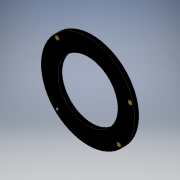
# Autodesk Inventor part: Neo_Cercle
Saved by Autodesk Inventor 2017 (Build 210142000, 142)
## iProperties
Created: 2018-11-03
Part Number: Neo_Cercle
Material: Generic
Document SubType Name: Modeling
Designer: ludov
Density: 1 g/cm^3
Appearance: Default
Author: ludov
Autodesk Inventor part; units mm, degrees
ref_plane "YZ Plane" through (0, 0, 0) normal (1, 0, 0) x (0, 1, 0)
ref_plane "XZ Plane" through (0, 0, 0) normal (0, 1, 0) x (-1, 0, 0)
ref_plane "XY Plane" through (0, 0, 0) normal (0, 0, 1) x (1, 0, 0)
sketch "Esquisse1" plane through (0, 0, 0) normal (0, 1, 0) x (-1, 0, 0)
  circle A0 centre (0, 0) radius 18.325
  dimension "d0" = 36.65
  constraints: 1 centre point, 1 coincident
  measures "d0" diameter of A0
extrude "Extrusion1" add sketch "Esquisse1" along normal blind 1.6
sketch "Esquisse2" plane through (0, 1.6, 0) normal (0, 1, 0) x (1, 0, 0)
  circle A0 centre (0, 0) radius 11.7
  dimension "d3" = 23.4
  constraints: 1 centre point, 1 coincident
  measures "d3" diameter of A0
hole "Perçage1" at (0, 1.6, 0) direction (0, -1, 0) diameter 23.4 end through all
sketch "Esquisse18" plane through (0, 1.6, 0) normal (0, 1, 0) x (1, 0, 0)
  line L0 (0, 0) -> (12.0738, 12.0738)
  line L1 (0, 0) -> (17.075, 0) construction
  circle A0 centre (12.0738, 12.0738) radius 0.8
  dimension "d116" = 17.075
  dimension "d117" = 45
  dimension "d118" = 1.6
  constraints: 4 end point, 1 centre point, 1 coincident, 1 equal length, 1 horizontal
  measures "d116" distance of L0.start L0.end
  measures "d117" angle of L1 L0
  measures "d118" diameter of A0
extrude "Extrusion14" add sketch "Esquisse18" along normal blind 0.05
sketch "Esquisse19" plane through (12.0738, 1.65, -12.0738) normal (0, 1, 0) x (1, 0, 0)
  circle A0 centre (0, 0) radius 0.45
  point P0 (-12.0738, -12.0738)
  dimension "d121" = 0.9
  constraints: 1 centre point
  measures "d121" diameter of A0
hole "Perçage2" at (12.0738, 1.65, -12.0738) direction (0, -1, 0) diameter 0.9 end through all
sketch "Esquisse20" plane through (0, 1.6, 0) normal (0, 1, 0) x (1, 0, 0)
  line L0 (0, 0) -> (16.4932, -4.4193)
  line L1 (0, 0) -> (17.075, 0) construction
  circle A0 centre (16.4932, -4.4193) radius 0.8
  dimension "d129" = 17.075
  dimension "d130" = 345
  dimension "d131" = 1.6
  constraints: 4 end point, 2 coincident, 1 centre point, 1 equal length, 1 horizontal
  measures "d129" distance of L0.start L0.end
  measures "d131" diameter of A0
extrude "Extrusion15" add sketch "Esquisse20" along normal blind 0.05
sketch "Esquisse21" plane through (16.4932, 1.65, 4.4193) normal (0, 1, 0) x (1, 0, 0)
  circle A0 centre (0, 0) radius 0.45
  point P0 (-16.4932, 4.4193)
  dimension "d134" = 0.9
  constraints: 1 centre point
  measures "d134" diameter of A0
hole "Perçage3" at (16.4932, 1.65, 4.4193) direction (0, -1, 0) diameter 0.9 end through all
sketch "Esquisse22" plane through (0, 1.6, 0) normal (0, 1, 0) x (1, 0, 0)
  line L0 (0, 0) -> (-12.0738, 12.0738)
  line L1 (0, 0) -> (17.075, 0) construction
  circle A0 centre (-12.0738, 12.0738) radius 0.8
  dimension "d142" = 17.075
  dimension "d143" = 135
  dimension "d144" = 1.6
  constraints: 4 end point, 2 coincident, 1 centre point, 1 equal length, 1 horizontal
  measures "d142" distance of L0.start L0.end
  measures "d143" angle of L1 L0
  measures "d144" diameter of A0
extrude "Extrusion16" add sketch "Esquisse22" along normal blind 0.05
sketch "Esquisse23" plane through (-12.0738, 1.65, -12.0738) normal (0, 1, 0) x (1, 0, 0)
  circle A0 centre (0, 0) radius 0.45
  point P0 (12.0738, -12.0738)
  dimension "d147" = 0.9
  constraints: 1 centre point
  measures "d147" diameter of A0
hole "Perçage4" at (-12.0738, 1.65, -12.0738) direction (0, -1, 0) diameter 0.9 end through all
sketch "Esquisse24" plane through (0, 1.6, 0) normal (0, 1, 0) x (1, 0, 0)
  line L0 (0, 0) -> (-12.0738, -12.0738)
  line L1 (0, 0) -> (17.075, 0) construction
  circle A0 centre (-12.0738, -12.0738) radius 0.8
  dimension "d155" = 17.075
  dimension "d156" = 225
  dimension "d157" = 1.6
  constraints: 4 end point, 2 coincident, 1 centre point, 1 equal length, 1 horizontal
  measures "d155" distance of L0.start L0.end
  measures "d157" diameter of A0
extrude "Extrusion17" add sketch "Esquisse24" along normal blind 0.05
sketch "Esquisse25" plane through (-12.0738, 1.65, 12.0738) normal (0, 1, 0) x (1, 0, 0)
  circle A0 centre (0, 0) radius 0.45
  point P0 (12.0738, 12.0738)
  dimension "d160" = 0.9
  constraints: 1 centre point
  measures "d160" diameter of A0
hole "Perçage5" at (-12.0738, 1.65, 12.0738) direction (0, -1, 0) diameter 0.9 end through all
sketch "Esquisse26" plane through (0, 1.6, 0) normal (0, 1, 0) x (1, 0, 0)
  line L0 (0, 0) -> (12.9577, 12.9577) construction
  circle A0 centre (0, 0) radius 18.325 projected
  line L1 (0, 0) -> (18.325, 0) construction
  line L2 (8.9166, 9.751) -> (10.8842, 11.7186) construction
  line L3 (10.8842, 11.7186) -> (11.6845, 10.9182) construction
  line L4 (11.6845, 10.9182) -> (9.7169, 8.9507) construction
  line L5 (9.7169, 8.9507) -> (8.9166, 9.751) construction
  spline S0 degree 2 poles (10.018, 9.3854) (9.9429, 9.3104) (9.7727, 9.2318) (9.6816, 9.2336) knots 0 0 0 1 2 2 2
  spline S1 degree 2 poles (9.6816, 9.2336) (9.5899, 9.2359) (9.4037, 9.327) (9.3137, 9.4169) knots 0 0 0 1 2 2 2
  spline S2 degree 2 poles (9.3137, 9.4169) (9.2283, 9.5023) (9.1412, 9.6857) (9.1378, 9.7785) knots 0 0 0 1 2 2 2
  spline S3 degree 2 poles (9.1378, 9.7785) (9.1344, 9.8679) (9.21, 10.0444) (9.2851, 10.1195) knots 0 0 0 1 2 2 2
  spline S4 degree 2 poles (9.2851, 10.1195) (9.3212, 10.1556) (9.3968, 10.2106) (9.4358, 10.2312) knots 0 0 0 1 2 2 2
  spline S5 degree 2 poles (9.4358, 10.2312) (9.4667, 10.2484) (9.5504, 10.2816) (9.5773, 10.2902) knots 0 0 0 1 2 2 2
  line L6 (9.5773, 10.2902) -> (9.6908, 10.1768)
  line L7 (9.6908, 10.1768) -> (9.6827, 10.1687)
  spline S6 degree 2 poles (9.6827, 10.1687) (9.6495, 10.1664) (9.5842, 10.1573) (9.5338, 10.1389) knots 0 0 0 1 2 2 2
  spline S7 degree 2 poles (9.5338, 10.1389) (9.4908, 10.1246) (9.398, 10.0696) (9.3555, 10.0272) knots 0 0 0 1 2 2 2
  spline S8 degree 2 poles (9.3555, 10.0272) (9.2536, 9.9252) (9.2811, 9.6456) (9.4088, 9.5178) knots 0 0 0 1 2 2 2
  spline S9 degree 2 poles (9.4088, 9.5178) (9.4799, 9.4467) (9.6197, 9.3734) (9.6879, 9.3682) knots 0 0 0 1 2 2 2
  spline S10 degree 2 poles (9.6879, 9.3682) (9.7549, 9.3619) (9.8793, 9.4095) (9.9332, 9.4633) knots 0 0 0 1 2 2 2
  spline S11 degree 2 poles (9.9332, 9.4633) (9.9727, 9.5029) (10.0403, 9.5934) (10.0558, 9.6318) knots 0 0 0 1 2 2 2
  line L8 (10.0558, 9.6318) -> (9.873, 9.8146)
  line L9 (9.873, 9.8146) -> (9.7091, 9.6507)
  line L10 (9.7091, 9.6507) -> (9.6266, 9.7332)
  line L11 (9.6266, 9.7332) -> (9.8833, 9.99)
  line L12 (9.8833, 9.99) -> (10.1922, 9.6811)
  spline S12 degree 2 poles (10.1922, 9.6811) (10.1824, 9.6553) (10.1463, 9.5699) (10.128, 9.5367) knots 0 0 0 1 2 2 2
  spline S13 degree 2 poles (10.128, 9.5367) (10.1033, 9.4914) (10.0575, 9.425) (10.018, 9.3854) knots 0 0 0 1 2 2 2
  line L13 (10.8632, 10.2581) -> (10.7577, 10.1527)
  line L14 (10.7577, 10.1527) -> (9.8352, 10.4495)
  line L15 (9.8352, 10.4495) -> (10.4449, 9.8398)
  line L16 (10.4449, 9.8398) -> (10.3572, 9.7521)
  line L17 (10.3572, 9.7521) -> (9.6501, 10.4593)
  line L18 (9.6501, 10.4593) -> (9.7836, 10.5928)
  line L19 (9.7836, 10.5928) -> (10.6282, 10.3177)
  line L20 (10.6282, 10.3177) -> (10.0684, 10.8776)
  line L21 (10.0684, 10.8776) -> (10.1561, 10.9652)
  line L22 (10.1561, 10.9652) -> (10.8632, 10.2581)
  spline S14 degree 2 poles (11.211, 11.3119) (11.3078, 11.2151) (11.3852, 10.9807) (11.3628, 10.8713) knots 0 0 0 1 2 2 2
  spline S15 degree 2 poles (11.3628, 10.8713) (11.3428, 10.7836) (11.2551, 10.6501) (11.1692, 10.5641) knots 0 0 0 1 2 2 2
  line L23 (11.1692, 10.5641) -> (11.0064, 10.4014)
  line L24 (11.0064, 10.4014) -> (10.2993, 11.1085)
  line L25 (10.2993, 11.1085) -> (10.4603, 11.2695)
  spline S16 degree 2 poles (10.4603, 11.2695) (10.56, 11.3692) (10.7033, 11.4529) (10.7698, 11.4666) knots 0 0 0 1 2 2 2
  spline S17 degree 2 poles (10.7698, 11.4666) (10.8832, 11.4895) (11.1078, 11.4151) (11.211, 11.3119) knots 0 0 0 1 2 2 2
  spline S18 degree 2 poles (11.1119, 11.2151) (11.0305, 11.2964) (10.8614, 11.3578) (10.7755, 11.3371) knots 0 0 0 1 2 2 2
  spline S19 degree 2 poles (10.7755, 11.3371) (10.7153, 11.3217) (10.6099, 11.2563) (10.5463, 11.1927) knots 0 0 0 1 2 2 2
  line L26 (10.5463, 11.1927) -> (10.4747, 11.1211)
  line L27 (10.4747, 11.1211) -> (11.019, 10.5767)
  line L28 (11.019, 10.5767) -> (11.0907, 10.6484)
  spline S20 degree 2 poles (11.0907, 10.6484) (11.1531, 10.7108) (11.2276, 10.8254) (11.2391, 10.8907) knots 0 0 0 1 2 2 2
  spline S21 degree 2 poles (11.2391, 10.8907) (11.2551, 10.9733) (11.1944, 11.1326) (11.1119, 11.2151) knots 0 0 0 1 2 2 2
  dimension "d168" = 45
  dimension "d170" = 0.59
  dimension "d182" = 13.2
  constraints: 4 end point, 1 equal length, 1 horizontal, 1 parallel, 4 other
  measures "d168" angle of L1 L0
  measures "d170" distance from line of L0 L2.start
  measures "d182" distance from line of L5 L0.start
emboss "Gravure1" sketch "Esquisse26" operation cut depth 0.02 direction (0, -1, 0) contours S0 S1 S2 S3 S4 S5 L6 L7 S6 S7 S8 S9 S10 S11 L8 L9 L10 L11 L12 S12 S13 | L13 L14 L15 L16 L17 L18 L19 L20 L21 L22 | S14 S15 L23 L24 L25 S16 S17
sketch "Esquisse27" plane through (0, 1.6, 0) normal (0, 1, 0) x (1, 0, 0)
  circle A0 centre (-12.0738, 12.0738) radius 0.8
  line L0 (-9.751, 8.9166) -> (-11.9316, 11.0972) construction
  line L1 (-11.9316, 11.0972) -> (-11.1836, 11.8452) construction
  line L2 (-11.1836, 11.8452) -> (-9.003, 9.6646) construction
  line L3 (-9.003, 9.6646) -> (-9.751, 8.9166) construction
  line L4 (0, 0) -> (-12.9518, 12.9518) construction
  line L5 (0, 0) -> (18.3166, 0) construction
  line L6 (-9.3619, 9.9417) -> (-9.088, 9.6678)
  line L7 (-9.088, 9.6678) -> (-9.1602, 9.5956)
  line L8 (-9.1602, 9.5956) -> (-9.2502, 9.6856)
  line L9 (-9.2502, 9.6856) -> (-9.8129, 9.1229)
  line L10 (-9.8129, 9.1229) -> (-9.7229, 9.0329)
  line L11 (-9.7229, 9.0329) -> (-9.7951, 8.9607)
  line L12 (-9.7951, 8.9607) -> (-10.069, 9.2346)
  line L13 (-10.069, 9.2346) -> (-9.9968, 9.3068)
  line L14 (-9.9968, 9.3068) -> (-9.9069, 9.2169)
  line L15 (-9.9069, 9.2169) -> (-9.3442, 9.7796)
  line L16 (-9.3442, 9.7796) -> (-9.4341, 9.8695)
  line L17 (-9.4341, 9.8695) -> (-9.3619, 9.9417)
  line L18 (-9.9842, 10.564) -> (-9.8788, 10.4586)
  line L19 (-9.8788, 10.4586) -> (-10.1756, 9.5361)
  line L20 (-10.1756, 9.5361) -> (-9.5659, 10.1457)
  line L21 (-9.5659, 10.1457) -> (-9.4782, 10.0581)
  line L22 (-9.4782, 10.0581) -> (-10.1854, 9.351)
  line L23 (-10.1854, 9.351) -> (-10.3189, 9.4845)
  line L24 (-10.3189, 9.4845) -> (-10.0438, 10.3291)
  line L25 (-10.0438, 10.3291) -> (-10.6037, 9.7693)
  line L26 (-10.6037, 9.7693) -> (-10.6913, 9.8569)
  line L27 (-10.6913, 9.8569) -> (-9.9842, 10.564)
  dimension "d180" = 135
  dimension "d183" = 13.2
  dimension "d186" = 0.59
  constraints: 4 end point, 1 centre point, 1 equal length, 1 horizontal, 2 other
  measures "d180" angle of L5 L4
  measures "d183" distance from line of L3 L4.start
  measures "d186" distance from line of L4 L0.start
emboss "Gravure2" sketch "Esquisse27" operation cut depth 0.02 direction (0, -1, 0) contours L6 L7 L8 L9 L10 L11 L12 L13 L14 L15 L16 L17 | L18 L19 L20 L21 L22 L23 L24 L25 L26 L27
sketch "Esquisse28" plane through (0, 1.6, 0) normal (0, 1, 0) x (1, 0, 0)
  circle A0 centre (-12.0738, -12.0738) radius 0.45 projected
  line L0 (0, 0) -> (-12.0738, -12.0738) construction
  line L1 (-11.7066, -10.8722) -> (-9.751, -8.9166) construction
  line L2 (-9.751, -8.9166) -> (-8.9903, -9.6773) construction
  line L3 (-8.9903, -9.6773) -> (-10.9459, -11.633) construction
  line L4 (-10.9459, -11.633) -> (-11.7066, -10.8722) construction
  spline S0 degree 2 poles (-11.0391, -10.3961) (-10.952, -10.4029) (-10.7697, -10.4958) (-10.6815, -10.584) knots 0 0 0 1 2 2 2
  spline S1 degree 2 poles (-10.6815, -10.584) (-10.5955, -10.67) (-10.4999, -10.8528) (-10.4941, -10.941) knots 0 0 0 1 2 2 2
  spline S2 degree 2 poles (-10.4941, -10.941) (-10.4884, -11.0338) (-10.5566, -11.196) (-10.6259, -11.2653) knots 0 0 0 1 2 2 2
  spline S3 degree 2 poles (-10.6259, -11.2653) (-10.6975, -11.337) (-10.8609, -11.4029) (-10.9502, -11.3971) knots 0 0 0 1 2 2 2
  spline S4 degree 2 poles (-10.9502, -11.3971) (-11.0379, -11.3908) (-11.2196, -11.2963) (-11.3067, -11.2092) knots 0 0 0 1 2 2 2
  spline S5 degree 2 poles (-11.3067, -11.2092) (-11.3955, -11.1204) (-11.4866, -10.941) (-11.4946, -10.8516) knots 0 0 0 1 2 2 2
  spline S6 degree 2 poles (-11.4946, -10.8516) (-11.5003, -10.7634) (-11.4339, -10.5995) (-11.3628, -10.5284) knots 0 0 0 1 2 2 2
  spline S7 degree 2 poles (-11.3628, -10.5284) (-11.2906, -10.4562) (-11.1244, -10.3909) (-11.0391, -10.3961) knots 0 0 0 1 2 2 2
  spline S8 degree 2 poles (-10.7795, -10.682) (-10.8494, -10.6121) (-10.9881, -10.5342) (-11.0511, -10.5261) knots 0 0 0 1 2 2 2
  spline S9 degree 2 poles (-11.0511, -10.5261) (-11.1158, -10.5175) (-11.2316, -10.56) (-11.2809, -10.6092) knots 0 0 0 1 2 2 2
  spline S10 degree 2 poles (-11.2809, -10.6092) (-11.3319, -10.6602) (-11.3731, -10.7725) (-11.3645, -10.8396) knots 0 0 0 1 2 2 2
  spline S11 degree 2 poles (-11.3645, -10.8396) (-11.3565, -10.9038) (-11.2774, -11.0424) (-11.2087, -11.1112) knots 0 0 0 1 2 2 2
  spline S12 degree 2 poles (-11.2087, -11.1112) (-11.0694, -11.2504) (-10.8047, -11.2814) (-10.7067, -11.1834) knots 0 0 0 1 2 2 2
  spline S13 degree 2 poles (-10.7067, -11.1834) (-10.6087, -11.0854) (-10.6402, -10.8212) (-10.7795, -10.682) knots 0 0 0 1 2 2 2
  spline S14 degree 2 poles (-9.9629, -10.6024) (-10.0254, -10.6648) (-10.1509, -10.725) (-10.2162, -10.725) knots 0 0 0 1 2 2 2
  spline S15 degree 2 poles (-10.2162, -10.725) (-10.2901, -10.7256) (-10.4236, -10.6528) (-10.4993, -10.5771) knots 0 0 0 1 2 2 2
  line L5 (-10.4993, -10.5771) -> (-10.9405, -10.1359)
  line L6 (-10.9405, -10.1359) -> (-10.8465, -10.0419)
  line L7 (-10.8465, -10.0419) -> (-10.4053, -10.4832)
  spline S16 degree 2 poles (-10.4053, -10.4832) (-10.356, -10.5324) (-10.2769, -10.5863) (-10.2323, -10.5955) knots 0 0 0 1 2 2 2
  spline S17 degree 2 poles (-10.2323, -10.5955) (-10.1847, -10.6052) (-10.0901, -10.5691) (-10.0432, -10.5221) knots 0 0 0 1 2 2 2
  spline S18 degree 2 poles (-10.0432, -10.5221) (-9.999, -10.478) (-9.9595, -10.38) (-9.9692, -10.3325) knots 0 0 0 1 2 2 2
  spline S19 degree 2 poles (-9.9692, -10.3325) (-9.9784, -10.2878) (-10.0317, -10.2093) (-10.0793, -10.1617) knots 0 0 0 1 2 2 2
  line L8 (-10.0793, -10.1617) -> (-10.5228, -9.7182)
  line L9 (-10.5228, -9.7182) -> (-10.4288, -9.6242)
  line L10 (-10.4288, -9.6242) -> (-9.9876, -10.0654)
  spline S20 degree 2 poles (-9.9876, -10.0654) (-9.9137, -10.1394) (-9.838, -10.2746) (-9.8397, -10.3485) knots 0 0 0 1 2 2 2
  spline S21 degree 2 poles (-9.8397, -10.3485) (-9.8403, -10.4155) (-9.8976, -10.537) (-9.9629, -10.6024) knots 0 0 0 1 2 2 2
  line L11 (-9.422, -10.0316) -> (-10.0454, -9.4082)
  line L12 (-10.0454, -9.4082) -> (-10.2827, -9.6454)
  line L13 (-10.2827, -9.6454) -> (-10.3663, -9.5617)
  line L14 (-10.3663, -9.5617) -> (-9.7979, -8.9933)
  line L15 (-9.7979, -8.9933) -> (-9.7142, -9.077)
  line L16 (-9.7142, -9.077) -> (-9.9515, -9.3142)
  line L17 (-9.9515, -9.3142) -> (-9.328, -9.9377)
  line L18 (-9.328, -9.9377) -> (-9.422, -10.0316)
  dimension "d187" = 0.59
  dimension "d188" = 13.2
  constraints: 2 end point, 1 parallel, 2 other
  measures "d187" distance from line of L0 L1.end
  measures "d188" distance from line of L2 L0.start
emboss "Gravure3" sketch "Esquisse28" operation cut depth 0.05 direction (0, -1, 0) contours S0 S1 S2 S3 S4 S5 S6 S7 | S14 S15 L5 L6 L7 S16 S17 S18 S19 L8 L9 L10 S20 S21 | L11 L12 L13 L14 L15 L16 L17 L18
sketch "Esquisse29" plane through (0, 1.6, 0) normal (0, 1, 0) x (1, 0, 0)
  line L0 (0, 0) -> (17.7006, -4.7429) construction
  circle A0 centre (0, 0) radius 18.325 projected
  line L1 (0, 0) -> (18.325, 0) construction
  line L2 (15.3486, -4.5371) -> (12.6441, -3.8124) construction
  line L3 (12.6441, -3.8124) -> (12.9029, -2.8465) construction
  line L4 (12.9029, -2.8465) -> (15.6075, -3.5712) construction
  line L5 (15.6075, -3.5712) -> (15.3486, -4.5371) construction
  spline S0 degree 2 poles (14.7183, -4.0561) (14.735, -3.9935) (14.8099, -3.8927) (14.8603, -3.8643) knots 0 0 0 1 2 2 2
  spline S1 degree 2 poles (14.8603, -3.8643) (14.9236, -3.8284) (15.0726, -3.8138) (15.176, -3.8415) knots 0 0 0 1 2 2 2
  line L6 (15.176, -3.8415) -> (15.2848, -3.8706)
  line L7 (15.2848, -3.8706) -> (15.3812, -3.5106)
  line L8 (15.3812, -3.5106) -> (15.5096, -3.545)
  line L9 (15.5096, -3.545) -> (15.2508, -4.5109)
  line L10 (15.2508, -4.5109) -> (15.0081, -4.4459)
  spline S2 degree 2 poles (15.0081, -4.4459) (14.922, -4.4228) (14.809, -4.3623) (14.7715, -4.3179) knots 0 0 0 1 2 2 2
  spline S3 degree 2 poles (14.7715, -4.3179) (14.7273, -4.2666) (14.6967, -4.1367) (14.7183, -4.0561) knots 0 0 0 1 2 2 2
  spline S4 degree 2 poles (14.8532, -4.0881) (14.8397, -4.1382) (14.8545, -4.221) (14.8834, -4.2539) knots 0 0 0 1 2 2 2
  spline S5 degree 2 poles (14.8834, -4.2539) (14.9085, -4.2824) (14.9855, -4.3207) (15.0457, -4.3368) knots 0 0 0 1 2 2 2
  line L11 (15.0457, -4.3368) -> (15.1522, -4.3654)
  line L12 (15.1522, -4.3654) -> (15.2554, -3.9802)
  line L13 (15.2554, -3.9802) -> (15.1677, -3.9567)
  spline S6 degree 2 poles (15.1677, -3.9567) (15.0895, -3.9358) (14.9865, -3.935) (14.9463, -3.9595) knots 0 0 0 1 2 2 2
  spline S7 degree 2 poles (14.9463, -3.9595) (14.9096, -3.9807) (14.8655, -4.0419) (14.8532, -4.0881) knots 0 0 0 1 2 2 2
  line L14 (13.4356, -4.0245) -> (13.937, -3.1236)
  line L15 (13.937, -3.1236) -> (14.0811, -3.1622)
  line L16 (14.0811, -3.1622) -> (14.0628, -4.0164)
  line L17 (14.0628, -4.0164) -> (14.4685, -3.266)
  line L18 (14.4685, -3.266) -> (14.611, -3.3042)
  line L19 (14.611, -3.3042) -> (14.5988, -4.3362)
  line L20 (14.5988, -4.3362) -> (14.4665, -4.3007)
  line L21 (14.4665, -4.3007) -> (14.4869, -3.448)
  line L22 (14.4869, -3.448) -> (14.0798, -4.1971)
  line L23 (14.0798, -4.1971) -> (13.9491, -4.1621)
  line L24 (13.9491, -4.1621) -> (13.972, -3.2999)
  line L25 (13.972, -3.2999) -> (13.5616, -4.0583)
  line L26 (13.5616, -4.0583) -> (13.4356, -4.0245)
  line L27 (12.8318, -2.8275) -> (12.9985, -2.8721)
  line L28 (12.9985, -2.8721) -> (13.2008, -3.3383)
  line L29 (13.2008, -3.3383) -> (13.348, -3.3777)
  line L30 (13.348, -3.3777) -> (13.451, -2.9934)
  line L31 (13.451, -2.9934) -> (13.5793, -3.0278)
  line L32 (13.5793, -3.0278) -> (13.3205, -3.9937)
  line L33 (13.3205, -3.9937) -> (13.0716, -3.927)
  spline S8 degree 2 poles (13.0716, -3.927) (12.9886, -3.9048) (12.8815, -3.8568) (12.8394, -3.8102) knots 0 0 0 1 2 2 2
  spline S9 degree 2 poles (12.8394, -3.8102) (12.7974, -3.7637) (12.7661, -3.6455) (12.7865, -3.5695) knots 0 0 0 1 2 2 2
  spline S10 degree 2 poles (12.7865, -3.5695) (12.8148, -3.4639) (12.9612, -3.3496) (13.0628, -3.3399) knots 0 0 0 1 2 2 2
  line L34 (13.0628, -3.3399) -> (12.8318, -2.8275)
  spline S11 degree 2 poles (12.9231, -3.5952) (12.9117, -3.6375) (12.9241, -3.7104) (12.9497, -3.74) knots 0 0 0 1 2 2 2
  spline S12 degree 2 poles (12.9497, -3.74) (12.9723, -3.7653) (13.0411, -3.7997) (13.0943, -3.8139) knots 0 0 0 1 2 2 2
  line L35 (13.0943, -3.8139) -> (13.2219, -3.8481)
  line L36 (13.2219, -3.8481) -> (13.3192, -3.4849)
  line L37 (13.3192, -3.4849) -> (13.2065, -3.4547)
  spline S13 degree 2 poles (13.2065, -3.4547) (13.1509, -3.4398) (13.0572, -3.4357) (13.0185, -3.4581) knots 0 0 0 1 2 2 2
  spline S14 degree 2 poles (13.0185, -3.4581) (12.9832, -3.4771) (12.9365, -3.5451) (12.9231, -3.5952) knots 0 0 0 1 2 2 2
  dimension "d191" = 15
  dimension "d196" = 0.59
  dimension "d197" = 13.2
  constraints: 4 end point, 1 equal length, 1 horizontal, 4 other
  measures "d191" angle of L0 L1
  measures "d196" distance from line of L0 L4.end
  measures "d197" distance from line of L3 L0.start
emboss "Gravure4" sketch "Esquisse29" operation cut depth 0.05 direction (0, -1, 0) contours S0 S1 L6 L7 L8 L9 L10 S2 S3 | L14 L15 L16 L17 L18 L19 L20 L21 L22 L23 L24 L25 L26 | L27 L28 L29 L30 L31 L32 L33 S8 S9 S10 L34
sketch "Esquisse30" plane through (0, 0, 0) normal (0, -1, 0) x (1, 0, 0)
  circle A0 centre (12.0738, -12.0738) radius 0.8 projected
  circle A1 centre (12.0738, -12.0738) radius 0.8
  point P0 (0, 0)
  constraints: 1 centre point, 1 coincident
extrude "Extrusion18" add sketch "Esquisse30" along normal blind 0.05
sketch "Esquisse31" plane through (12.0738, -0.05, -12.0738) normal (0, -1, 0) x (1, 0, 0)
  circle A0 centre (0, 0) radius 0.45
  point P0 (-12.0738, 12.0738)
  dimension "d200" = 0.9
  constraints: 1 centre point
  measures "d200" diameter of A0
hole "Perçage6" at (12.0738, -0.05, -12.0738) direction (0, 1, 0) diameter 0.9 end through all
sketch "Esquisse32" plane through (0, 0, 0) normal (0, -1, 0) x (1, 0, 0)
  circle A0 centre (16.4932, 4.4193) radius 0.8 projected
  circle A1 centre (16.4932, 4.4193) radius 0.8
  point P0 (0, 0)
  dimension "d208" = 1.6
  constraints: 1 centre point, 1 coincident
  measures "d208" diameter of A1
extrude "Extrusion19" add sketch "Esquisse32" along normal blind 0.05
sketch "Esquisse33" plane through (16.4932, -0.05, 4.4193) normal (0, -1, 0) x (1, 0, 0)
  circle A0 centre (0, 0) radius 0.45
  point P0 (-16.4932, -4.4193)
  dimension "d211" = 0.9
  constraints: 1 centre point
  measures "d211" diameter of A0
hole "Perçage7" at (16.4932, -0.05, 4.4193) direction (0, 1, 0) diameter 0.9 end through all
sketch "Esquisse34" plane through (0, 0, 0) normal (0, -1, 0) x (1, 0, 0)
  circle A0 centre (-12.0738, 12.0738) radius 0.45 projected
  circle A1 centre (-12.0738, 12.0738) radius 0.8
  point P0 (0, 0)
  dimension "d219" = 1.6
  constraints: 1 centre point, 1 coincident
  measures "d219" diameter of A1
extrude "Extrusion20" add sketch "Esquisse34" along normal blind 0.05
